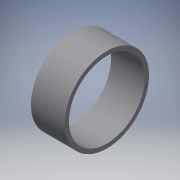
# Autodesk Inventor part: NASA-20-WT-01
Saved by Autodesk Inventor 2019 (Build 230136000, 136)
## iProperties
Created: 2019-09-05
Part Number: NASA-20-WT-01
Material: ABS Plastic
Document SubType Name: Modeling
Designer: Rick Szalay
Density: 1.06 g/cm^3
Appearance: Smooth - Red
Author: Rick Szalay
Autodesk Inventor part; units mm, degrees
ref_plane "YZ Plane" through (0, 0, 0) normal (1, 0, 0) x (0, 1, 0)
ref_plane "XZ Plane" through (0, 0, 0) normal (0, 1, 0) x (-1, 0, 0)
ref_plane "XY Plane" through (0, 0, 0) normal (0, 0, 1) x (1, 0, 0)
sketch "Sketch1" plane through (0, 0, 0) normal (1, 0, 0) x (0, 1, 0)
  circle A0 centre (0, 0) radius 114.3
  circle A1 centre (0, 0) radius 127
  dimension "d0" = 228.6
  dimension "d1" = 254
  constraints: 2 centre point, 1 coincident
  measures "d0" diameter of A0
  measures "d1" diameter of A1
extrude "Extrusion1" add sketch "Sketch1" along normal blind 82.55 and the other way blind 19.05
body "Solid1"
